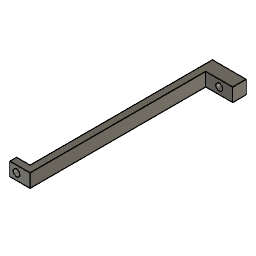
stand frame (Autodesk Fusion 360 design; units mm, degrees)
part number: 2026-02-28-00-57-03-953
Autodesk Fusion 360 part; units mm, degrees
sketch "Sketch1" plane through (0, 0, 0) normal (0, 0, 1) x (1, 0, 0)
  line L0 (0, 0) -> (0, 260)
  line L1 (0, 0) -> (-30, 0)
  line L2 (-30, 0) -> (0, 0)
  line L3 (0, 0) -> (0, 10)
  line L4 (0, 10) -> (-30, 10)
  line L5 (-30, 10) -> (-30, 0)
  line L6 (0, 10) -> (-10, 10)
  line L7 (-10, 10) -> (-10, 280)
  line L8 (-10, 280) -> (40, 280)
  line L9 (40, 280) -> (40, 260)
  line L10 (40, 260) -> (-10, 260)
  line L11 (-10, 260) -> (-10, 280)
  dimension "d1" = 260
  dimension "d2" = 30
  dimension "d3" = 10
  dimension "d4" = 270
  dimension "d5" = 50
  dimension "d6" = 20
  constraint coincident L0.start L1.start
  constraint vertical L0
  constraint perpendicular L0 L1
  constraint horizontal L2
  constraint vertical L3
  constraint horizontal L4
  constraint vertical L5
  constraint coincident L4 L6.end
  constraint perpendicular L6 L7
  constraint horizontal L8
  constraint vertical L9
  constraint horizontal L10
  constraint vertical L11
  measures "d1" distance of L0.start L0.end
  measures "d2" distance of L0.start L1.end
  measures "d3" distance of L1.end L4.end
  measures "d4" distance of L6.end L7.end
  measures "d5" distance of L7.end L8.end
  measures "d6" distance of L7.end L10.end
extrude "Extrude1" add sketch "Sketch1" along normal blind 20
sketch "Sketch2" plane through (0, 260, 0) normal (0, -1, 0) x (1, 0, 0)
  line L0 (0, 0) -> (40, 0)
  line L1 (40, 0) -> (40, 20)
  line L2 (40, 20) -> (0, 20)
  line L3 (0, 20) -> (0, 0)
  line L4 (20, 20) -> (20, 10)
  circle A0 centre (20, 10) radius 5
  dimension "d9" = 10
  constraint midpoint L2 L4.start
  constraint perpendicular L2 L4
  constraint coincident L4.end A0.centre
  measures "d9" diameter of A0
sketch "Sketch3" plane through (0, 10, 0) normal (0, 1, 0) x (-1, 0, 0)
  line L0 (10, 0) -> (30, 0)
  line L1 (30, 0) -> (30, 20)
  line L2 (30, 20) -> (10, 20)
  line L3 (10, 20) -> (10, 0)
  circle A0 centre (20, 10) radius 5
  dimension "d10" = 10
  measures "d10" diameter of A0
extrude "Extrude2" cut sketch "Sketch3" against normal blind 25 contours A0
extrude "Extrude3" cut sketch "Sketch2" against normal blind 100 contours A0
